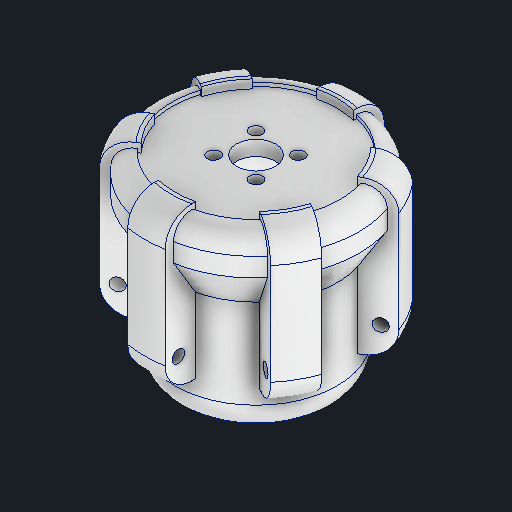
# Autodesk Inventor part: Corredor
Saved by Autodesk Inventor 2025.3 (Build 293356030, 356C)
## iProperties
Created: 2024-11-15
Part Number: Corredor
Material: Aluminio 6061
Document SubType Name: Modeling
Designer: j.santaa
Density: 2.7 g/cm^3
Appearance: Aluminio - Plano
Mass: 46.3771 g
Surface Area: 199.886 cm^2
Volume: 46.3771 cm^3
Author: j.santaa
Autodesk Inventor part; units mm, degrees
ref_plane "YZ Plane" through (0, 0, 0) normal (1, 0, 0) x (0, 1, 0)
sketch "Sketch4" plane through (0, 0, 0) normal (1, 0, 0) x (0, 1, 0)
  line L0 (5.2, 0) -> (18.425, 0)
  line L1 (18.425, 0) -> (18.425, -45)
  line L2 (0, 5) -> (0, -45)
  line L3 (5.2, 0) -> (5.2, 5)
  line L4 (5.2, 5) -> (27.5, 5)
  line L5 (27.5, 5) -> (27.5, -5)
  line L6 (27.5, -5) -> (21.7125, -14.6727)
  line L7 (21.7125, -14.6727) -> (21.7125, -45)
  line L8 (21.7125, -45) -> (18.425, -45)
  point P0 (0, 0)
  point P1 (24.25, -5)
  dimension "d11" = 36.85
  dimension "d12" = 10.4
  dimension "d13" = 5
  dimension "d14" = 10
  dimension "d15" = 55
  dimension "d18" = 3.25
  dimension "d19" = 10
  dimension "d22" = 43.425
  dimension "d59" = 50
  constraints: 18 end point, 4 horizontal alignment, 4 vertical, 2 perpendicular, 1 horizontal, 1 point on line
  measures "d11" diameter of L1 L2
  measures "d12" diameter of L3 L2
  measures "d13" distance of L0.start L3.end
  measures "d14" distance of L4.end L5.end
  measures "d15" diameter of L5 L2
  measures "d18" distance of L5.end point (24.25, -5)
  measures "d19" distance of L6.end point (24.25, -5)
  measures "d22" diameter of L7 L2
  measures "d59" distance between parallel lines of L8 L4
revolve "Revolution2" add sketch "Sketch4" angle 360 about axis through (0, 0, 5) along (0, 0, -1)
ref_plane "Work Plane1" through (0, 0, -19.682) normal (0, 0, 1) x (1, 0, 0)
sketch "Sketch5" plane through (0, 0, -19.682) normal (0, 0, 1) x (1, 0, 0)
  arc A0 (-29.2888, 5) -> (-29.2888, -5) centre (0, 0) ccw
  line L0 (-29.2888, 5) -> (-21.129, 5)
  line L1 (-29.2888, -5) -> (-21.129, -5)
  circle A1 centre (0, 0) radius 21.7125 projected
  point P0 (-29.7125, 0)
  point P1 (-21.7125, 0)
  dimension "Dedos" = 10
  dimension "d72" = 8
  constraints: 6 point on circle, 4 end point, 2 horizontal alignment, 1 centre point, 1 coincident, 1 concentric, 1 horizontal, 1 parallel
  measures "Dedos" distance between parallel lines of L1 L0
  measures "d72" distance of point (-29.713, 0) point (-21.712, 0)
extrude "Extrusion1" add sketch "Sketch5" against normal blind 15 contours L0 A1 L1 A0
ref_plane "Work Plane2" through (-29.2888, 0, -19.682) normal (0, -1, 0) x (1, 0, 0)
sketch "Sketch7" plane through (-29.2888, 0, -19.682) normal (0, -1, 0) x (1, 0, 0)
  line L0 (-0.4237, 0) -> (-0.4237, -15) projected
  circle A0 centre (3.5488, -7.5) radius 1.5
  line L1 (7.5763, -25.318) -> (51.0013, -25.318) projected
  line L2 (29.2888, -25.318) -> (29.2888, 24.682) construction
  line L3 (24.0888, 24.682) -> (34.4888, 24.682) projected
  point P0 (29.2888, 19.682)
  point P1 (-0.4237, -7.5)
  dimension "d45" = 3
  dimension "d83" = 25.74
  constraints: 3 midpoint, 2 end point, 1 centre point, 1 coincident, 1 horizontal alignment
  measures "d45" diameter of A0
  measures "d83" distance from line of L2 A0.centre
fillet "Fillet2" radius 7 1 edges at (-29.7125, 0, -34.682)
pattern_circular "Circular Pattern1" count 6 over 360 about axis through (0, 0, -29.8363) along (0, 0, -1) of "Extrusion1", "Fillet2"
fillet "Fillet3" radius 8 1 edges at (0, -21.7125, -45)
fillet "Fillet3" radius 5 1 edges at (0, -27.5, 5)
sketch "Sketch8" plane through (0, 0, 5) normal (0, 0, 1) x (1, 0, 0)
  line L0 (-5.657, -5.657) -> (5.657, -5.657) construction
  line L1 (5.657, -5.657) -> (5.657, 5.657) construction
  line L2 (5.657, 5.657) -> (-5.657, 5.657) construction
  line L3 (-5.657, 5.657) -> (-5.657, -5.657) construction
  line L4 (-5.657, -5.657) -> (5.657, 5.657) construction
  line L5 (5.657, -5.657) -> (-5.657, 5.657) construction
  point P0 (0, 0)
  dimension "d51" = 11.314
  constraints: 12 end point, 4 coincident, 2 midpoint, 2 parallel, 2 perpendicular, 1 horizontal
  measures "d51" distance of L2.end L0.start
hole "Hole2" at (-5.657, -5.657, 5) at (-5.657, 5.657, 5) at (5.657, 5.657, 5) at (5.657, -5.657, 5) direction (0, 0, -1) diameter 3.4 end through all clearance for "Countersunk Flat Head Screw ISO 2009/7046" size "M3" standard "ISO"
sketch "Boceto10" plane through (21.129, 5, -19.682) normal (0, 0, 1) x (1, 0, 0)
  line L0 (8.1598, 0) -> (0, 0) projected
  arc A0 (0, -10) -> (0, 0) centre (-21.129, -5) ccw projected
  line L1 (0, -10) -> (8.1598, -10) projected
  arc A1 (8.1598, -10) -> (8.1598, 0) centre (-21.129, -5) ccw projected
  point P0 (-21.129, -5)
extrude "Extrusión3" add sketch "Boceto10" along normal blind 26
fillet "Empalme4" radius 7 1 edges at (29.7125, 0, 6.318)
pattern_circular "Patrón circular2" count 6 over 360 about axis through (0, 0, -29.8363) along (0, 0, -1) of "Empalme4", "Extrusión3"
sketch "Boceto11" plane through (0, 0, 5) normal (0, 0, 1) x (1, 0, 0)
  arc A0 (6.6386, 21.4984) -> (-6.6386, 21.4984) centre (0, 0) ccw projected
  circle A1 centre (0, 0) radius 5.2 projected
  circle A2 centre (-5.657, -5.657) radius 1.7 projected
  circle A3 centre (-5.657, 5.657) radius 1.7 projected
  circle A4 centre (5.657, 5.657) radius 1.7 projected
  circle A5 centre (5.657, -5.657) radius 1.7 projected
  line L0 (6.2343, 20.7982) -> (6.6386, 21.4984) projected
  line L1 (-6.6386, 21.4984) -> (-6.2343, 20.7982) projected
  arc A6 (-6.2343, 20.7982) -> (-14.8946, 15.7982) centre (0, 0) ccw projected
  line L2 (-14.8946, 15.7982) -> (-15.2988, 16.4984) projected
  arc A7 (-15.2988, 16.4984) -> (-21.9374, 5) centre (0, 0) ccw projected
  line L3 (-21.9374, 5) -> (-21.129, 5) projected
  arc A8 (-21.129, 5) -> (-21.129, -5) centre (0, 0) ccw projected
  line L4 (-21.129, -5) -> (-21.9374, -5) projected
  arc A9 (-21.9374, -5) -> (-15.2988, -16.4984) centre (0, 0) ccw projected
  line L5 (-15.2988, -16.4984) -> (-14.8946, -15.7982) projected
  arc A10 (-14.8946, -15.7982) -> (-6.2343, -20.7982) centre (0, 0) ccw projected
  line L6 (-6.2343, -20.7982) -> (-6.6386, -21.4984) projected
  arc A11 (-6.6386, -21.4984) -> (6.6386, -21.4984) centre (0, 0) ccw projected
  line L7 (6.6386, -21.4984) -> (6.2343, -20.7982) projected
  arc A12 (6.2343, -20.7982) -> (14.8946, -15.7982) centre (0, 0) ccw projected
  line L8 (14.8946, -15.7982) -> (15.2988, -16.4984) projected
  arc A13 (15.2988, -16.4984) -> (21.9374, -5) centre (0, 0) ccw projected
  line L9 (21.9374, -5) -> (21.129, -5) projected
  arc A14 (21.129, -5) -> (21.129, 5) centre (0, 0) ccw projected
  line L10 (21.129, 5) -> (21.9374, 5) projected
  arc A15 (21.9374, 5) -> (15.2988, 16.4984) centre (0, 0) ccw projected
  line L11 (15.2988, 16.4984) -> (14.8946, 15.7982) projected
  arc A16 (14.8946, 15.7982) -> (6.2343, 20.7982) centre (0, 0) ccw projected
  point P0 (0, 0)
extrude "Extrusión4" cut sketch "Boceto11" against normal blind 1
sketch "Boceto12" plane through (-21.129, 5, -14.6727) normal (0, 1, 0) x (1, 0, 0)
  point P0 (-4.611, 12.5093)
hole "Agujero3" at (-25.74, 5, -27.182) direction (0, -1, 0) diameter 3.4 end through all clearance for "Tornillo de cabeza plana avellanada ISO 2009/7046" size "M3" standard "ISO"
pattern_circular "Patrón circular3" count 6 over 360 about axis through (0, 0, -29.8363) along (0, 0, -1) of "Agujero3"
body "Solid2"
